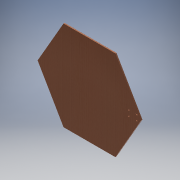
# Autodesk Inventor part: BA015
Saved by Autodesk Inventor 2017 (Build 210142000, 142)
## iProperties
Created: 2018-10-18
Part Number: BA015
Material: Wood (Oak)
Document SubType Name: Modeling
Designer: Dell
Density: 0.76 g/cm^3
Appearance: White Oak - Natural Medium Gloss
Author: Dell
Autodesk Inventor part; units mm, degrees
ref_plane "YZ Plane" through (0, 0, 0) normal (1, 0, 0) x (0, 1, 0)
ref_plane "XZ Plane" through (0, 0, 0) normal (0, 1, 0) x (-1, 0, 0)
ref_plane "XY Plane" through (0, 0, 0) normal (0, 0, 1) x (1, 0, 0)
sketch "Sketch1" plane through (0, 0, 0) normal (0, 0, 1) x (1, 0, 0)
  line L0 (146.05, 252.966) -> (292.1, 0)
  line L1 (292.1, 0) -> (146.05, -252.966)
  line L2 (146.05, -252.966) -> (-146.05, -252.966)
  line L3 (-146.05, -252.966) -> (-292.1, 0)
  line L4 (-292.1, 0) -> (-146.05, 252.966)
  line L5 (-146.05, 252.966) -> (146.05, 252.966)
  point P0 (0, 0)
  point P1 (0, 0)
  dimension "d3" = 584.2
  constraints: 12 end point, 1 coincident, 1 horizontal alignment, 13 other
  measures "d3" distance of L0.end L3.end
extrude "Extrusion1" add sketch "Sketch1" along normal blind 6.35
sketch "Sketch7" plane through (0, 0, 6.35) normal (0, 0, 1) x (1, 0, 0)
  line L0 (292.1, 0) -> (146.05, 252.966) projected
  line L1 (146.05, 252.966) -> (-146.05, 252.966) projected
  line L2 (-146.05, 252.966) -> (-292.1, 0) projected
  line L3 (-292.1, 0) -> (-146.05, -252.966) projected
  line L4 (-146.05, -252.966) -> (146.05, -252.966) projected
  line L5 (146.05, -252.966) -> (292.1, 0) projected
  line L6 (-299.4323, 0) -> (-149.7162, 259.316)
  line L7 (-149.7162, 259.316) -> (149.7162, 259.316)
  line L8 (149.7162, 259.316) -> (299.4323, 0)
  line L9 (299.4323, 0) -> (149.7162, -259.316)
  line L10 (149.7162, -259.316) -> (-149.7162, -259.316)
  line L11 (-149.7162, -259.316) -> (-299.4323, 0)
  point P0 (0, 0)
  dimension "d20" = 6.35
  constraints: 12 end point, 5 other
  measures "d20" distance between parallel lines of L2 L6
extrude "Extrusion7" add sketch "Sketch7" against normal blind 6.35
sketch "Sketch8" plane through (0, 0, 6.35) normal (0, 0, 1) x (1, 0, 0)
  arc A0 (274.0293, -21.5946) -> (279.0293, -16.5946) centre (274.0293, -16.5946) ccw
  line L0 (279.0293, -16.5946) -> (279.0293, 16.2054)
  arc A1 (279.0293, 16.2054) -> (274.0293, 21.2054) centre (274.0293, 16.2054) ccw
  line L1 (274.0293, 21.2054) -> (224.2293, 21.2054)
  arc A2 (224.2293, 21.2054) -> (219.2293, 16.2054) centre (224.2293, 16.2054) ccw
  line L2 (219.2293, 16.2054) -> (219.2293, -16.5946)
  arc A3 (219.2293, -16.5946) -> (224.2293, -21.5946) centre (224.2293, -16.5946) ccw
  line L3 (224.2293, -21.5946) -> (274.0293, -21.5946)
  arc A4 (273.3793, -18.3946) -> (273.3793, -12.2946) centre (273.3793, -15.3446) ccw
  line L4 (270.4793, -18.3946) -> (273.3793, -18.3946)
  arc A5 (270.4793, -12.2946) -> (270.4793, -18.3946) centre (270.4793, -15.3446) ccw
  line L5 (273.3793, -12.2946) -> (270.4793, -12.2946)
  arc A6 (273.3793, 11.9054) -> (273.3793, 18.0054) centre (273.3793, 14.9554) ccw
  line L6 (270.4793, 11.9054) -> (273.3793, 11.9054)
  arc A7 (270.4793, 18.0054) -> (270.4793, 11.9054) centre (270.4793, 14.9554) ccw
  line L7 (273.3793, 18.0054) -> (270.4793, 18.0054)
  arc A8 (224.8793, 18.0054) -> (224.8793, 11.9054) centre (224.8793, 14.9554) ccw
  line L8 (227.7793, 18.0054) -> (224.8793, 18.0054)
  arc A9 (227.7793, 11.9054) -> (227.7793, 18.0054) centre (227.7793, 14.9554) ccw
  line L9 (224.8793, 11.9054) -> (227.7793, 11.9054)
  arc A10 (224.8793, -12.2946) -> (224.8793, -18.3946) centre (224.8793, -15.3446) ccw
  line L10 (227.7793, -12.2946) -> (224.8793, -12.2946)
  arc A11 (227.7793, -18.3946) -> (227.7793, -12.2946) centre (227.7793, -15.3446) ccw
  line L11 (224.8793, -18.3946) -> (227.7793, -18.3946)
  point P0 (0, 0)
  point P1 (249.1293, -0.1946)
  constraints: 24 end point, 24 point on circle, 12 centre point
extrude "Extrusion8" cut sketch "Sketch8" against normal blind 6.35 contours L4 A5 L5 A4 | L6 A7 L7 A6 | L8 A9 L9 A8 | L10 A11 L11 A10
body "Solid1"
